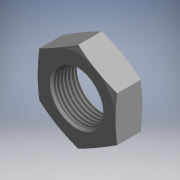
# Autodesk Inventor part: DIN-439-B - M22x1.5(F)
Saved by Autodesk Inventor 2017.3 (Build 213256000, 256)
## iProperties
Part Number: DIN-439-B - M22x1.5(F)
Material: Generic
Catalog Web Link: www.cadenas.de
Description: DIN-439 Form B-Hex nut
Vendor: FESTO
Document SubType Name: Modeling
Designer: partserver
Manufacturer: FESTO
Mass: 6.08938 g
Surface Area: 29.3855 cm^2
Volume: 6.08938 cm^3
Density: 1 g/cm^3
Appearance: PSOLRGB-192-192-192
Category: PARTsolutions
Company: FESTO
Title: DIN-439-B - M22x1.5
Author: Cadenas PARTsolutions
Comments: Hex nut
PSOL_IDENT_0: {$CADENAS_DATA\23d-libs\festo\zyl_zubeh\din_439_b\din_439_form_b.prj},190 {VTYP=3D},{NB=DIN-439-B -
PSOL_IDENT_1: M22x1.5(F)},{LINA=DIN-439-B - M22x1.5},{NN=DIN-439 Form B},{DATE=28.05.2015 11:05:12},{GEOMDATE=28.0
PSOL_IDENT_2: 5.2015 08:07:00},{VERSION=},{LINEID=400},{WBVAR=},{WBNUMERIC=}  {NB=DIN-439-B - M22x1.5(F)},{LINA=DI
PSOL_IDENT_3: N-439-B - M22x1.5},{KT=X},{IDNR=},{NENN=M22x1.5},{DG=22.000},{DK=20.376},{M=11.000},{S=32.000},{P=1.
PSOL_IDENT_4: 500}
NB: DIN-439-B - M22x1.5(F)
NN: DIN-439 Form B
NT: Hex nut
NBSYN: DIN-439-B - $NENN.(F)
LINA: DIN-439-B - M22x1.5
CATALOG: Festo
ROWDESC: M22x1.5
NENN: M22x1.5
DG: 22
DK: 20.376
M: 11
S: 32
P: 1.5
SUPPLIER: FESTO
ARTICLENO: DIN-439-B - M22x1.5(F)
BOMINFO: DIN-439-B - M22x1.5
CREATOR: CADENAS GmbH
Autodesk Inventor part; units mm, degrees
sketch "Sketch_1" plane through (0, 0, 0) normal (0, 0, 1) x (1, 0, 0)
  line L0 (0, -11) -> (0, 0)
  line L1 (0, 0) -> (15.95, 0)
  line L2 (15.95, 0) -> (36.4763, -5.5)
  line L3 (36.4763, -5.5) -> (15.95, -11)
  line L4 (15.95, -11) -> (0, -11)
  line L5 (0, -11) -> (0, 0)
  constraints: 12 end point
revolve "Revolution1" add sketch "Sketch_1" angle 360 about axis through (0, -11, 0) along (0, 1, 0)
sketch "Sketch_2" plane through (0, 0, 0) normal (0, 1, 0) x (-1, 0, 0)
  line L0 (64, -64) -> (64, 64)
  line L1 (64, 64) -> (-64, 64)
  line L2 (-64, 64) -> (-64, -64)
  line L3 (-64, -64) -> (64, -64)
  line L4 (16, 9.2376) -> (0, 18.4752)
  line L5 (0, 18.4752) -> (-16, 9.2376)
  line L6 (-16, 9.2376) -> (-16, -9.2376)
  line L7 (-16, -9.2376) -> (0, -18.4752)
  line L8 (0, -18.4752) -> (16, -9.2376)
  line L9 (16, -9.2376) -> (16, 9.2376)
  constraints: 20 end point
extrude "Extrusion1" cut sketch "Sketch_2" along normal mid plane 24
sketch "Sketch_3" plane through (0, 0, 0) normal (0, 0, 1) x (1, 0, 0)
  line L0 (0, -11) -> (0, 0)
  line L1 (0, 0) -> (11, 0)
  line L2 (11, 0) -> (10.188, -0.812)
  line L3 (10.188, -0.812) -> (10.188, -10.188)
  line L4 (10.188, -10.188) -> (11, -11)
  line L5 (11, -11) -> (0, -11)
  line L6 (0, -11) -> (0, 0)
  constraints: 14 end point
revolve "Revolution2" cut sketch "Sketch_3" angle 360 about axis through (0, -11, 0) along (0, -1, 0)
thread "Thread1" size "M22x1.5" class "6H" standard "ISO Metric profile" full length
ref_plane "2CYL_XY" through (0, -5.5, 0) normal (0, 1, 0) x (1, 0, 0)
ref_plane "2CYL_YZ" through (0, -5.5, 0) normal (1, 0, 0) x (0, 0, -1)
ref_plane "2CYL_ZX" through (0, -5.5, 0) normal (0, 0, -1) x (0, 1, 0)
ref_plane "din439b_punkt_XY" through (0, 0, 0) normal (0, 1, 0) x (1, 0, 0)
ref_plane "din439b_punkt_YZ" through (0, 0, 0) normal (1, 0, 0) x (0, 0, -1)
ref_plane "din439b_punkt_ZX" through (0, 0, 0) normal (0, 0, -1) x (0, 1, 0)
body "Solid1"
